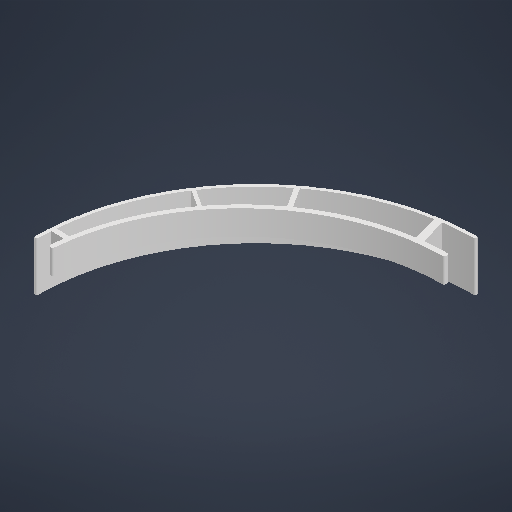
# Autodesk Inventor part: HalfFilterwall2.5
Saved by Autodesk Inventor 2026 (Build 300175050, 175E)
## iProperties
Created: 2026-05-09
Part Number: HalfFilterwall2.5
Material: Generic
Document SubType Name: Modeling
Designer: sniel
Density: 1 g/cm^3
Appearance: Default
Author: sniel
Autodesk Inventor part; units mm, degrees
ref_plane "YZ Plane" through (0, 0, 0) normal (1, 0, 0) x (0, 1, 0)
ref_plane "XZ Plane" through (0, 0, 0) normal (0, 1, 0) x (-1, 0, 0)
ref_plane "XY Plane" through (0, 0, 0) normal (0, 0, 1) x (1, 0, 0)
sketch "Sketch1" plane through (0, 0, 0) normal (0, 1, 0) x (-1, 0, 0)
  line L0 (25.911358, 34.249133) -> (21.233221, 33.384269)
  arc A0 (20.051555, 34.383526) -> (21.233221, 33.384269) centre (21.051429, 34.367606) ccw
  arc A1 (-119.771311, -90.200681) -> (-23.872169, 132.589761) centre (-107.167892, 36.409132) ccw
  arc A2 (26.72784, 35.291188) -> (-23.872169, 132.589761) centre (-107.276076, 27.409132) ccw
  arc A3 (25.911358, 34.249133) -> (26.72784, 35.291188) centre (25.729565, 35.23247) ccw
  line L1 (27.846781, 45.663576) -> (26.350119, 52.659387)
  arc A4 (26.262284, 53.120201) -> (26.350119, 52.659387) centre (31.458205, 53.871804) ccw
  line L2 (26.262284, 53.120201) -> (25.087055, 60.131828)
  arc A5 (25.087055, 60.131828) -> (9.491125, 97.783734) centre (-107.160239, 27.409181) ccw
  line L3 (9.491125, 97.783734) -> (5.313504, 103.677111)
  arc A6 (5.078674, 104.022902) -> (5.313504, 103.677111) centre (9.535809, 106.797148) ccw
  line L4 (5.078674, 104.022902) -> (1.211947, 109.965755)
  arc A7 (1.211947, 109.965755) -> (-24.603666, 135.781367) centre (-107.160239, 27.409181) ccw
  line L5 (-24.603666, 135.781367) -> (-30.7027, 139.78928)
  arc A8 (-30.976063, 139.975227) -> (-30.7027, 139.78928) centre (-27.88806, 144.221018) ccw
  line L6 (-30.976063, 139.975227) -> (-36.785686, 144.060546)
  arc A9 (-36.785686, 144.060546) -> (-74.437592, 159.656476) centre (-107.160239, 27.409181) ccw
  line L7 (-74.437592, 159.656476) -> (-81.696835, 160.968275)
  arc A10 (-81.90007, 161.007105) -> (-81.696835, 160.968275) centre (-80.813404, 166.143413) ccw
  line L8 (-81.90007, 161.007105) -> (-88.905844, 162.416202)
  arc A11 (-88.905844, 162.416202) -> (-106.269539, 163.641796) centre (-107.160239, 27.409181) ccw
  arc A12 (-106.269539, 163.641796) -> (-107.276076, 162.641817) centre (-106.276076, 162.641817) ccw
  line L9 (-107.276076, 162.641817) -> (-107.276076, 162.640681)
  arc A13 (-107.276076, 162.640681) -> (-106.28403, 161.640713) centre (-106.276076, 162.640681) ccw
  arc A14 (-107.276076, -87.826394) -> (-106.28403, 161.640713) centre (-107.276076, 36.909132) ccw
  arc A15 (17.1741, 28.476759) -> (18.171813, 27.409157) centre (18.171813, 28.409157) ccw
  line L10 (18.171813, 27.409157) -> (18.813932, 27.409157)
  arc A16 (18.813932, 27.409157) -> (19.811922, 28.345783) centre (18.813932, 28.409157) ccw
  arc A17 (19.811922, 28.345783) -> (19.924171, 30.367744) centre (-107.167892, 36.409132) ccw
  arc A18 (20.745107, 31.304304) -> (19.924171, 30.367744) centre (20.923043, 30.320262) ccw
  line L11 (20.745107, 31.304304) -> (25.726971, 32.205131)
  arc A19 (26.904498, 31.249699) -> (25.726971, 32.205131) centre (25.904907, 31.221089) ccw
  arc A20 (26.955779, 28.401762) -> (26.904498, 31.249699) centre (-107.276076, 27.409132) ccw
  arc A21 (26.955779, 28.401762) -> (27.955752, 27.409157) centre (27.955752, 28.409157) ccw
  line L12 (27.955752, 27.409157) -> (28.071589, 27.409157)
  arc A22 (28.071589, 27.409157) -> (29.071562, 28.416551) centre (28.071589, 28.409157) ccw
  arc A23 (29.071562, 28.416551) -> (27.846781, 45.663576) centre (-107.160605, 27.409157) ccw
  circle A24 centre (-80.813404, -111.325149) radius 5.25
  circle A25 centre (-27.88806, -89.402754) radius 5.25
  circle A26 centre (31.458205, 0.94646) radius 5.25
  circle A27 centre (9.535809, -51.978884) radius 5.25
  line L13 (-36.901523, -89.242233) -> (-34.200843, -93.452293)
  arc A28 (-34.200843, -93.452293) -> (-21.799144, -85.023816) centre (-27.88806, -89.402754) ccw
  line L14 (-21.799144, -85.023816) -> (-24.719503, -80.963054)
  arc A29 (-24.719503, -80.963054) -> (1.09611, -55.147441) centre (-107.276076, 27.409132) ccw
  line L15 (1.09611, -55.147441) -> (5.156872, -58.067801)
  arc A30 (5.156872, -58.067801) -> (13.585349, -45.666101) centre (9.535809, -51.978884) ccw
  line L16 (13.585349, -45.666101) -> (9.375288, -42.965421)
  arc A31 (9.375288, -42.965421) -> (24.971218, -5.313515) centre (-107.276076, 27.409132) ccw
  line L17 (24.971218, -5.313515) -> (29.85785, -6.380809)
  arc A32 (29.85785, -6.380809) -> (32.667342, 8.348351) centre (31.458205, 0.94646) ccw
  line L18 (32.667342, 8.348351) -> (27.730944, 9.154737)
  arc A33 (27.730944, 9.154737) -> (28.95945, 27.409132) centre (-107.276076, 27.409132) ccw
  line L19 (28.95945, 27.409132) -> (26.95945, 27.409132)
  arc A34 (-107.276076, -106.826394) -> (26.95945, 27.409132) centre (-107.276076, 27.409132) ccw
  line L20 (-107.276076, -106.826394) -> (-107.276076, -108.826394)
  arc A35 (-107.276076, -108.826394) -> (-89.021681, -107.597889) centre (-107.276076, 27.409132) ccw
  line L21 (-89.021681, -107.597889) -> (-88.215295, -112.534287)
  arc A36 (-88.215295, -112.534287) -> (-73.486136, -109.724794) centre (-80.813404, -111.325149) ccw
  line L22 (-73.486136, -109.724794) -> (-74.553429, -104.838163)
  arc A37 (-74.553429, -104.838163) -> (-36.901523, -89.242233) centre (-107.276076, 27.409132) ccw
  arc A38 (-242.283097, 45.663527) -> (-241.384565, 3.429309) centre (-107.276076, 27.409132) ccw
  arc A39 (-240.795426, 0.340666) -> (-241.384565, 3.429309) centre (-246.010358, 0.94646) ccw
  arc A40 (-240.795426, 0.340666) -> (-220.82881, -47.863009) centre (-107.276076, 27.409132) ccw
  arc A41 (-219.061393, -50.463594) -> (-220.82881, -47.863009) centre (-224.087962, -51.978884) ccw
  arc A42 (-219.061393, -50.463594) -> (-185.148803, -84.376185) centre (-107.276076, 27.409132) ccw
  arc A43 (-182.548218, -86.143602) -> (-185.148803, -84.376185) centre (-186.664093, -89.402754) ccw
  arc A44 (-182.548218, -86.143602) -> (-134.344543, -106.110218) centre (-107.276076, 27.409132) ccw
  arc A45 (-131.255899, -106.699356) -> (-134.344543, -106.110218) centre (-133.738749, -111.325149) ccw
  arc A46 (-131.255899, -106.699356) -> (-107.276076, -108.826394) centre (-107.276076, 27.409132) ccw
  line L23 (-107.276076, -108.826394) -> (-107.276076, -106.826394)
  arc A47 (-121.457864, -106.075149) -> (-107.276076, -106.826394) centre (-107.276076, 27.409132) ccw
  arc A48 (-123.445042, -105.849042) -> (-121.457864, -106.075149) centre (-107.276076, 27.409132) ccw
  arc A49 (-157.822596, -96.946109) -> (-123.445042, -105.849042) centre (-107.276076, 27.409132) ccw
  arc A50 (-159.669726, -96.179225) -> (-157.822596, -96.946109) centre (-107.276076, 27.409132) ccw
  arc A51 (-206.235704, -63.289096) -> (-159.669726, -96.179225) centre (-107.276076, 27.409132) ccw
  arc A52 (-207.576012, -61.804652) -> (-206.235704, -63.289096) centre (-107.276076, 27.409132) ccw
  arc A53 (-239.250006, 2.872252) -> (-207.576012, -61.804652) centre (-107.276076, 27.409132) ccw
  line L24 (-239.250006, 2.872252) -> (-207.929881, 9.417778)
  arc A54 (-207.65189, 3.035935) -> (-207.929881, 9.417778) centre (-239.600927, 4.841225) ccw
  arc A55 (-207.65189, 3.035935) -> (-188.343026, -44.330718) centre (-112.100514, 14.368223) ccw
  line L25 (-188.343026, -44.330718) -> (-207.576012, -61.804652)
  line L26 (-207.576012, -61.804652) -> (-206.235704, -63.289096)
  line L27 (-206.235704, -63.289096) -> (-186.045327, -47.222959)
  arc A56 (-186.045327, -47.222959) -> (-151.387404, -76.230271) centre (-92.212994, 29.679581) ccw
  line L28 (-151.387404, -76.230271) -> (-159.669726, -96.179225)
  line L29 (-159.669726, -96.179225) -> (-157.822596, -96.946109)
  line L30 (-157.822596, -96.946109) -> (-149.623192, -77.196874)
  arc A57 (-149.623192, -77.196874) -> (-121.536367, -88.043175) centre (-92.212994, 29.679581) ccw
  line L31 (-121.536367, -88.043175) -> (-123.445042, -105.849042)
  line L32 (-123.445042, -105.849042) -> (-121.457864, -106.075149)
  line L33 (-121.457864, -106.075149) -> (-119.591748, -88.510568)
  arc A58 (-119.591748, -88.510568) -> (-107.276076, -90.701527) centre (-92.212994, 29.679581) ccw
  line L34 (-107.276076, -90.701527) -> (-107.276076, -87.691339)
  arc A59 (-186.12244, -42.313227) -> (-107.276076, -87.691339) centre (-90.976951, 31.817552) ccw
  arc A60 (-206.317087, 11.782837) -> (-186.12244, -42.313227) centre (-103.213586, 19.455019) ccw
  arc A61 (-206.317087, 11.782837) -> (-242.283097, 45.663527) centre (-244.886371, 6.869839) ccw
  line L35 (-107.276076, -87.826394) -> (-107.276076, -106.826394)
  line L36 (26.95945, 27.409132) -> (17.097158, 27.409132)
  line L37 (26.672343, 18.634321) -> (18.872207, 19.008431)
  line L38 (18.872207, 19.008431) -> (18.426921, 16.041661)
  line L39 (18.426921, 16.041661) -> (26.444031, 15.657145)
  line L40 (16.478066, -24.59172) -> (6.890528, -19.978524)
  line L41 (6.890528, -19.978524) -> (5.52939, -22.651968)
  line L42 (5.52939, -22.651968) -> (15.284432, -27.345761)
  line L43 (-7.681148, -62.591016) -> (-16.709117, -53.067685)
  line L44 (-16.709117, -53.067685) -> (-18.843827, -55.17553)
  line L45 (-18.843827, -55.17553) -> (-9.721365, -64.798539)
  line L46 (-101.531289, -90.701527) -> (-101.531289, -106.70341)
  line L47 (-101.531289, -106.70341) -> (-98.535659, -106.541536)
  line L48 (-98.535659, -106.541536) -> (-98.535659, -90.533278)
  point P0 (0, 0)
  point P1 (19.748974, 27.409132)
  point P2 (-107.276076, -90.701527)
  point P3 (-107.276076, -90.826394)
  point P4 (-107.276076, -90.701527)
  dimension "d0" = 3
  dimension "d1" = 3
  dimension "d2" = 3
  dimension "d3" = 3
  constraints: 114 point on circle, 98 end point, 60 centre point, 4 parallel, 2 point on line, 2 vertical, 1 horizontal, 26 other
  measures "d0" distance of L37.end L38.end
  measures "d1" distance of L40.end L41.end
  measures "d2" distance of L43.end L44.end
  measures "d3" distance of L46.end L47.end
extrude "Extrusion1" add sketch "Sketch1" along normal blind 30 contours A1 L35 L34 A14 L36 L10 L38 L41 L44 | A34 L19 L12 A33 L18 A32 L17 A31 L16 A30 L15 A29 L14 A28 L13 A37 L22 A36 L21 A35 L20 | L44 A1 | L41 A1 | L38 A1 | A1 L37 A34 L39
sketch "Sketch2" plane through (0, 30, 0) normal (0, 1, 0) x (1, 0, 0)
  arc A0 (-26.672343, -18.634321) -> (-26.95945, -27.409132) centre (107.276076, -27.409132) ccw
  line L0 (-26.672343, -18.634321) -> (-18.872207, -19.008431)
  arc A1 (-18.872207, -19.008431) -> (-19.748974, -27.409132) centre (107.167892, -36.409132) ccw
  line L1 (-19.748974, -27.409132) -> (-17.097158, -27.409132)
  arc A2 (107.276076, 87.826394) -> (-17.097158, -27.409132) centre (107.276076, -36.909132) ccw
  line L2 (107.276076, 87.826394) -> (107.276076, 90.826394)
  arc A3 (107.276076, 90.826394) -> (-18.426921, -16.041661) centre (107.167892, -36.409132) ccw
  line L3 (-18.426921, -16.041661) -> (-26.444031, -15.657145)
  arc A4 (107.276076, 106.826394) -> (-26.444031, -15.657145) centre (107.276076, -27.409132) ccw
  line L4 (107.276076, 106.826394) -> (107.276076, 108.826394)
  arc A5 (107.276076, 108.826394) -> (89.021681, 107.597889) centre (107.276076, -27.409132) ccw
  line L5 (89.021681, 107.597889) -> (88.215295, 112.534287)
  arc A6 (88.215295, 112.534287) -> (73.486136, 109.724794) centre (80.813404, 111.325149) ccw
  line L6 (73.486136, 109.724794) -> (74.553429, 104.838163)
  arc A7 (74.553429, 104.838163) -> (36.901523, 89.242233) centre (107.276076, -27.409132) ccw
  line L7 (36.901523, 89.242233) -> (34.200843, 93.452293)
  arc A8 (34.200843, 93.452293) -> (21.799144, 85.023816) centre (27.88806, 89.402754) ccw
  line L8 (21.799144, 85.023816) -> (24.719503, 80.963054)
  arc A9 (24.719503, 80.963054) -> (-1.09611, 55.147441) centre (107.276076, -27.409132) ccw
  line L9 (-1.09611, 55.147441) -> (-5.156872, 58.067801)
  arc A10 (-5.156872, 58.067801) -> (-13.585349, 45.666101) centre (-9.535809, 51.978884) ccw
  line L10 (-13.585349, 45.666101) -> (-9.375288, 42.965421)
  arc A11 (-9.375288, 42.965421) -> (-24.971218, 5.313515) centre (107.276076, -27.409132) ccw
  line L11 (-24.971218, 5.313515) -> (-29.85785, 6.380809)
  arc A12 (-29.85785, 6.380809) -> (-32.667342, -8.348351) centre (-31.458205, -0.94646) ccw
  line L12 (-32.667342, -8.348351) -> (-27.730944, -9.154737)
  arc A13 (-27.730944, -9.154737) -> (-28.95945, -27.409132) centre (107.276076, -27.409132) ccw
  line L13 (-28.95945, -27.409132) -> (-26.95945, -27.409132)
  circle A14 centre (-9.535809, 51.978884) radius 5.25
  circle A15 centre (-31.458205, -0.94646) radius 5.25
  circle A16 centre (27.88806, 89.402754) radius 5.25
  circle A17 centre (80.813404, 111.325149) radius 5.25
  line L14 (84.25805, 104.838163) -> (88.187372, 89.402754)
  line L15 (88.178618, 105.460968) -> (92.963712, 90.031099)
  line L16 (24.719503, 78.437874) -> (32.366834, 66.516533)
  line L17 (26.786511, 80.018082) -> (34.482298, 68.021204)
  line L18 (-5.325819, 45.666101) -> (4.808569, 39.165069)
  line L19 (-4.230022, 47.327515) -> (6.006369, 40.76105)
  point P0 (0, 0)
  constraints: 12 end point, 12 point on circle, 2 parallel
extrude "Extrusion2" add sketch "Sketch2" against normal blind 30 contours A3 L14 A4 L15 | A3 L16 A4 L17 | A3 L18 A4 L19
fillet "Fillet1" radius 1 8 edges at (-28.9594, 15, 27.4091) (-26.9594, 15, 27.4091) (-17.0972, 15, 27.4091) (-19.749, 15, 27.4091) (107.2761, 15, -87.8264) (107.2761, 15, -90.8264) (107.2761, 15, -106.8264) (107.2761, 15, -108.8264)
sketch "Sketch3" plane through (0, 0, 0) normal (0, -1, 0) x (1, 0, 0)
  arc A0 (106.268682, -108.822669) -> (106.283471, -106.822724) centre (106.276076, -107.822697) ccw
  arc A1 (88.178618, -105.460968) -> (106.283471, -106.822724) centre (107.276076, 27.409132) ccw
  line L0 (88.178618, -105.460968) -> (92.963712, -90.031099)
  arc A2 (92.963712, -90.031099) -> (106.269012, -90.823265) centre (107.167892, 36.409132) ccw
  arc A3 (106.269012, -90.823265) -> (107.276076, -89.82329) centre (106.276076, -89.82329) ccw
  line L1 (107.276076, -88.822417) -> (107.276076, -89.82329)
  arc A4 (107.276076, -88.822417) -> (106.28403, -87.822449) centre (106.276076, -88.822417) ccw
  arc A5 (-17.023755, 26.492641) -> (106.28403, -87.822449) centre (107.276076, 36.909132) ccw
  arc A6 (-17.023755, 26.492641) -> (-18.020262, 27.409132) centre (-18.020262, 26.409132) ccw
  line L2 (-18.670972, 27.409132) -> (-18.020262, 27.409132)
  arc A7 (-18.670972, 27.409132) -> (-19.667829, 26.329915) centre (-18.670972, 26.409132) ccw
  arc A8 (-19.667829, 26.329915) -> (-18.872207, 19.008431) centre (107.167892, 36.409132) ccw
  line L3 (-26.672343, 18.634321) -> (-18.872207, 19.008431)
  arc A9 (-26.95578, 26.416526) -> (-26.672343, 18.634321) centre (107.276076, 27.409132) ccw
  arc A10 (-26.95578, 26.416526) -> (-28.955725, 26.401737) centre (-27.955752, 26.409132) ccw
  arc A11 (-28.955725, 26.401737) -> (-27.730944, 9.154737) centre (107.276076, 27.409132) ccw
  line L4 (-32.667342, 8.348351) -> (-27.730944, 9.154737)
  arc A12 (-32.667342, 8.348351) -> (-29.85785, -6.380809) centre (-31.458205, 0.94646) ccw
  line L5 (-24.971218, -5.313515) -> (-29.85785, -6.380809)
  arc A13 (-24.971218, -5.313515) -> (-9.375288, -42.965421) centre (107.276076, 27.409132) ccw
  line L6 (-13.585349, -45.666101) -> (-9.375288, -42.965421)
  arc A14 (-13.585349, -45.666101) -> (-5.156872, -58.067801) centre (-9.535809, -51.978884) ccw
  line L7 (-1.09611, -55.147441) -> (-5.156872, -58.067801)
  arc A15 (-1.09611, -55.147441) -> (24.719503, -80.963054) centre (107.276076, 27.409132) ccw
  line L8 (21.799144, -85.023816) -> (24.719503, -80.963054)
  arc A16 (21.799144, -85.023816) -> (34.200843, -93.452293) centre (27.88806, -89.402754) ccw
  line L9 (36.901523, -89.242233) -> (34.200843, -93.452293)
  arc A17 (36.901523, -89.242233) -> (74.553429, -104.838163) centre (107.276076, 27.409132) ccw
  line L10 (73.486136, -109.724794) -> (74.553429, -104.838163)
  arc A18 (73.486136, -109.724794) -> (88.215295, -112.534287) centre (80.813404, -111.325149) ccw
  line L11 (89.021681, -107.597889) -> (88.215295, -112.534287)
  arc A19 (89.021681, -107.597889) -> (106.268682, -108.822669) centre (107.276076, 27.409132) ccw
  arc A20 (6.006369, -40.76105) -> (32.366834, -66.516533) centre (107.167892, 36.409132) ccw
  line L12 (32.366834, -66.516533) -> (24.719503, -78.437874)
  arc A21 (-4.230022, -47.327515) -> (24.719503, -78.437874) centre (107.276076, 27.409132) ccw
  line L13 (-4.230022, -47.327515) -> (6.006369, -40.76105)
  line L14 (88.187372, -89.402754) -> (84.25805, -104.838163)
  arc A22 (26.786511, -80.018082) -> (84.25805, -104.838163) centre (107.276076, 27.409132) ccw
  line L15 (26.786511, -80.018082) -> (34.482298, -68.021204)
  arc A23 (34.482298, -68.021204) -> (88.187372, -89.402754) centre (107.167892, 36.409132) ccw
  line L16 (4.808569, -39.165069) -> (-5.325819, -45.666101)
  arc A24 (-26.444031, 15.657145) -> (-5.325819, -45.666101) centre (107.276076, 27.409132) ccw
  line L17 (-18.426921, 16.041661) -> (-26.444031, 15.657145)
  arc A25 (-18.426921, 16.041661) -> (4.808569, -39.165069) centre (107.167892, 36.409132) ccw
  circle A26 centre (-9.535809, -51.978884) radius 5.25
  circle A27 centre (-31.458205, 0.94646) radius 5.25
  circle A28 centre (27.88806, -89.402754) radius 5.25
  circle A29 centre (80.813404, -111.325149) radius 5.25
  circle A30 centre (107.276076, 27.409132) radius 134.235526
  point P0 (0, 0)
  point P1 (-26.444031, 15.657145)
  point P2 (-4.230022, -47.327515)
  constraints: 1 coincident, 3 other
extrude "Extrusion3" cut sketch "Sketch3" against normal blind 15 contours A30 L14 A23 L15 L12 A20 L13 L16 A25 L17 L3 A8 A7 L2 A6 A5 A4 L1 A3 A2 L0
sketch "Sketch4" plane through (0, 30, 0) normal (0, 1, 0) x (1, 0, 0)
  arc A0 (106.283471, 106.822724) -> (106.268682, 108.822669) centre (106.276076, 107.822697) ccw
  arc A1 (106.268682, 108.822669) -> (89.021681, 107.597889) centre (107.276076, -27.409132) ccw
  line L0 (89.021681, 107.597889) -> (88.215295, 112.534287)
  arc A2 (88.215295, 112.534287) -> (73.486136, 109.724794) centre (80.813404, 111.325149) ccw
  line L1 (73.486136, 109.724794) -> (74.553429, 104.838163)
  arc A3 (74.553429, 104.838163) -> (36.901523, 89.242233) centre (107.276076, -27.409132) ccw
  line L2 (36.901523, 89.242233) -> (34.200843, 93.452293)
  arc A4 (34.200843, 93.452293) -> (21.799144, 85.023816) centre (27.88806, 89.402754) ccw
  line L3 (21.799144, 85.023816) -> (24.719503, 80.963054)
  arc A5 (24.719503, 80.963054) -> (-1.09611, 55.147441) centre (107.276076, -27.409132) ccw
  line L4 (-1.09611, 55.147441) -> (-5.156872, 58.067801)
  arc A6 (-5.156872, 58.067801) -> (-13.585349, 45.666101) centre (-9.535809, 51.978884) ccw
  line L5 (-13.585349, 45.666101) -> (-9.375288, 42.965421)
  arc A7 (-9.375288, 42.965421) -> (-24.971218, 5.313515) centre (107.276076, -27.409132) ccw
  line L6 (-24.971218, 5.313515) -> (-29.85785, 6.380809)
  arc A8 (-29.85785, 6.380809) -> (-32.667342, -8.348351) centre (-31.458205, -0.94646) ccw
  line L7 (-32.667342, -8.348351) -> (-27.730944, -9.154737)
  arc A9 (-27.730944, -9.154737) -> (-28.955725, -26.401737) centre (107.276076, -27.409132) ccw
  arc A10 (-28.955725, -26.401737) -> (-26.95578, -26.416526) centre (-27.955752, -26.409132) ccw
  arc A11 (-26.672343, -18.634321) -> (-26.95578, -26.416526) centre (107.276076, -27.409132) ccw
  line L8 (-26.672343, -18.634321) -> (-18.872207, -19.008431)
  arc A12 (-18.872207, -19.008431) -> (-19.667829, -26.329915) centre (107.167892, -36.409132) ccw
  arc A13 (-19.667829, -26.329915) -> (-18.670972, -27.409132) centre (-18.670972, -26.409132) ccw
  line L9 (-18.670972, -27.409132) -> (-18.020262, -27.409132)
  arc A14 (-18.020262, -27.409132) -> (-17.023755, -26.492641) centre (-18.020262, -26.409132) ccw
  arc A15 (106.28403, 87.822449) -> (-17.023755, -26.492641) centre (107.276076, -36.909132) ccw
  arc A16 (106.28403, 87.822449) -> (107.276076, 88.822417) centre (106.276076, 88.822417) ccw
  line L10 (107.276076, 88.822417) -> (107.276076, 89.82329)
  arc A17 (107.276076, 89.82329) -> (106.269012, 90.823265) centre (106.276076, 89.82329) ccw
  arc A18 (106.269012, 90.823265) -> (92.963712, 90.031099) centre (107.167892, -36.409132) ccw
  line L11 (92.963712, 90.031099) -> (88.178618, 105.460968)
  arc A19 (106.283471, 106.822724) -> (88.178618, 105.460968) centre (107.276076, -27.409132) ccw
  arc A20 (88.187372, 89.402754) -> (34.482298, 68.021204) centre (107.167892, -36.409132) ccw
  line L12 (34.482298, 68.021204) -> (26.786511, 80.018082)
  arc A21 (84.25805, 104.838163) -> (26.786511, 80.018082) centre (107.276076, -27.409132) ccw
  line L13 (84.25805, 104.838163) -> (88.187372, 89.402754)
  arc A22 (4.808569, 39.165069) -> (-18.426921, -16.041661) centre (107.167892, -36.409132) ccw
  line L14 (-18.426921, -16.041661) -> (-26.444031, -15.657145)
  arc A23 (-5.325819, 45.666101) -> (-26.444031, -15.657145) centre (107.276076, -27.409132) ccw
  line L15 (-5.325819, 45.666101) -> (4.808569, 39.165069)
  line L16 (6.006369, 40.76105) -> (-4.230022, 47.327515)
  arc A24 (24.719503, 78.437874) -> (-4.230022, 47.327515) centre (107.276076, -27.409132) ccw
  line L17 (24.719503, 78.437874) -> (32.366834, 66.516533)
  arc A25 (32.366834, 66.516533) -> (6.006369, 40.76105) centre (107.167892, -36.409132) ccw
  circle A26 centre (-9.535809, 51.978884) radius 5.25
  circle A27 centre (-31.458205, -0.94646) radius 5.25
  circle A28 centre (27.88806, 89.402754) radius 5.25
  circle A29 centre (80.813404, 111.325149) radius 5.25
  circle A30 centre (107.276076, -27.409132) radius 136.235526
  point P0 (0, 0)
  point P1 (-26.832412, -3.429309)
  point P2 (-26.243273, -0.340666)
  point P3 (-24.971218, 5.313515)
  point P4 (-6.276657, 47.863009)
  point P5 (-4.50924, 50.463594)
  point P6 (29.40335, 84.376185)
  point P7 (32.003935, 86.143602)
  point P8 (36.901523, 89.242233)
  point P9 (80.20761, 106.110218)
  point P10 (83.296254, 106.699356)
  point P11 (89.021681, 107.597889)
  constraints: 1 coincident, 3 other
extrude "Extrusion4" cut sketch "Sketch4" against normal blind 20 contours A30 A29 L1 A2 L0 | L7 A8 L6 A30 A27 | A30 A28 L3 A4 L2 | L5 A6 L4 A30 A26
body "Solid1"
